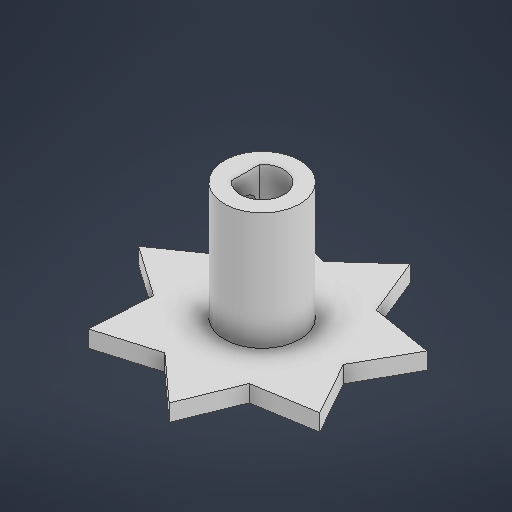
# Autodesk Inventor part: gear
Saved by Autodesk Inventor 2026.2 (Build 302298000, 298)
## iProperties
Created: 2026-04-06
Part Number: gear
Material: Generic
Document SubType Name: Modeling
Designer: Brian Wang
Density: 1 g/cm^3
Appearance: Default
Author: Brian Wang
Autodesk Inventor part; units mm, degrees
ref_plane "YZ Plane" through (0, 0, 0) normal (1, 0, 0) x (0, 1, 0)
ref_plane "XZ Plane" through (0, 0, 0) normal (0, 1, 0) x (-1, 0, 0)
ref_plane "XY Plane" through (0, 0, 0) normal (0, 0, 1) x (1, 0, 0)
sketch "Sketch1" plane through (0, 0, 0) normal (0, 1, 0) x (-1, 0, 0)
  line L0 (7.3724, 5.1622) -> (14.7447, 0)
  line L1 (14.7447, 0) -> (7.3724, -5.1622)
  line L2 (0.5606, 8.9825) -> (9.1932, 11.5279)
  line L3 (9.1932, 11.5279) -> (8.6326, 2.5454)
  line L4 (-6.6733, 6.0388) -> (-3.281, 14.3751)
  line L5 (-3.281, 14.3751) -> (3.3923, 8.3362)
  line L6 (-8.8821, -1.4522) -> (-13.2845, 6.3975)
  line L7 (-13.2845, 6.3975) -> (-4.4025, 7.8497)
  line L8 (-4.4025, -7.8497) -> (-13.2845, -6.3975)
  line L9 (-13.2845, -6.3975) -> (-8.8821, 1.4522)
  line L10 (3.3923, -8.3362) -> (-3.281, -14.3751)
  line L11 (-3.281, -14.3751) -> (-6.6733, -6.0388)
  line L12 (8.6326, -2.5454) -> (9.1932, -11.5279)
  line L13 (9.1932, -11.5279) -> (0.5606, -8.9825)
  arc A0 (-6.6733, -6.0388) -> (-5.3444, -7.2414) centre (0, 0) ccw
  arc A1 (7.3724, -5.1622) -> (7.957, -4.2054) centre (0, 0) ccw
  arc A2 (8.2491, -3.599) -> (8.6326, -2.5454) centre (0, 0) ccw
  point P0 (-6.0457, -7.5811)
  point P1 (2.1577, -9.4534)
  point P2 (8.7363, -4.2072)
  point P3 (8.7363, 4.2072)
  point P4 (2.1577, 9.4534)
  point P5 (-6.0457, 7.5811)
  point P6 (-9.6965, 0)
  dimension "d5" = 360
  constraints: 28 end point, 6 point on circle, 3 centre point, 3 point on line, 1 coincident, 36 other
extrude "Extrusion1" add sketch "Sketch1" along normal blind 2
sketch "Sketch2" plane through (0, 2, 0) normal (0, 1, 0) x (1, 0, 0)
  circle A0 centre (0, 0) radius 4.5
  dimension "d9" = 9
  constraints: 1 centre point, 1 coincident
  measures "d9" diameter of A0
extrude "Extrusion2" add sketch "Sketch2" along normal blind 14
sketch "Sketch3" plane through (0, 16, 0) normal (0, 1, 0) x (1, 0, 0)
  arc A0 (-1.976, -1.6898) -> (-1.976, 1.6898) centre (0, 0) ccw
  line L0 (-1.976, -1.6898) -> (-1.976, 1.6898)
  line L1 (2.6, 0) -> (2.6, 18.1631)
  dimension "d19" = 2.6
  constraints: 4 end point, 3 point on circle, 2 vertical, 1 centre point, 1 coincident, 1 tangent
  measures "d19" radius of A0
extrude "Extrusion3" cut sketch "Sketch3" against normal through all
sketch "Sketch4" plane through (-1.976, 16, 1.6898) normal (1, 0, 0) x (0, 0, -1)
  circle A0 centre (1.6248, -3.7675) radius 1.35
  point P0 (1.6898, -16)
  dimension "d16" = 2.7
  constraints: 1 centre point
  measures "d16" diameter of A0
extrude "Extrusion4" cut sketch "Sketch4" against normal blind 10
body "Solid1"
